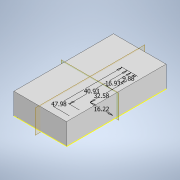
# Autodesk Inventor part: Micro-controller mount
Saved by Autodesk Inventor 2021 (Build 250183000, 183)
## iProperties
Created: 2020-08-19
Part Number: Micro-controller mount
Material: Generic
Document SubType Name: Modeling
Designer: zackh
Density: 1 g/cm^3
Appearance: Default
Author: zackh
Autodesk Inventor part; units mm, degrees
ref_plane "YZ Plane" through (0, 0, 0) normal (1, 0, 0) x (0, 1, 0)
ref_plane "XZ Plane" through (0, 0, 0) normal (0, 1, 0) x (-1, 0, 0)
ref_plane "XY Plane" through (0, 0, 0) normal (0, 0, 1) x (1, 0, 0)
sketch "Sketch1" plane through (0, 0, 0) normal (0, 1, 0) x (-1, 0, 0)
  line L0 (0, 0) -> (37, 0)
  line L1 (37, 0) -> (37, -70)
  line L2 (37, -70) -> (0, -70)
  line L3 (0, -70) -> (0, 0)
  dimension "d0" = 70
  dimension "d1" = 37
  constraints: 8 end point, 2 parallel, 1 horizontal, 1 perpendicular
  measures "d0" distance of L0.end L1.end
  measures "d1" distance of L1.end L2.end
extrude "Extrusion1" add sketch "Sketch1" along normal blind 15
sketch "Sketch2" plane through (0, 0, 0) normal (0, -1, 0) x (1, 0, 0)
  line L0 (-37, 0) -> (0, 0) projected
  line L1 (-18.5, 0) -> (-18.5, -70) construction
  line L2 (0, -70) -> (-37, -70) projected
  line L3 (0, 0) -> (0, -70) projected
  line L4 (0, -35) -> (-37, -35) construction
  line L5 (-37, -70) -> (-37, 0) projected
  line L6 (-2.28, 0) -> (-2.28, -70) construction
  line L7 (-34.72, 0) -> (-34.72, -70) construction
  line L8 (0, -67.58) -> (-35, -67.58) construction
  line L9 (0, -2.42) -> (-35, -2.42) construction
  line L10 (0, -57.7) -> (-35, -57.7) construction
  line L11 (0, -50.65) -> (-35, -50.65) construction
  line L12 (0, -26.65) -> (-35, -26.65) construction
  line L13 (0, -19.6) -> (-35, -19.6) construction
  point P0 (-17.5, -57.7)
  point P1 (-17.5, -50.65)
  point P2 (-17.5, -26.65)
  point P3 (-17.5, -19.6)
  dimension "d4" = 16.22
  dimension "d5" = 32.58
  dimension "d6" = 9.88
  dimension "d7" = 16.93
  dimension "d8" = 40.93
  dimension "d9" = 47.98
  constraints: 20 end point, 8 midpoint, 6 parallel, 4 symmetric about line
  measures "d4" distance between parallel lines of L1 L6
  measures "d5" distance between parallel lines of L4 L8
  measures "d6" distance between parallel lines of L8 L10
  measures "d7" distance between parallel lines of L8 L11
  measures "d8" distance between parallel lines of L8 L12
  measures "d9" distance between parallel lines of L8 L13
hole "Hole1" at (-17.5, 0, -57.7) at (-17.5, 0, -26.65) direction (0, 1, 0) diameter 2.459 depth 10 tip angle 118 thread size "M3x0.5" class "6H" standard "ANSI Metric M Profile"
hole "Hole2" at (-17.5, 0, -50.65) at (-17.5, 0, -19.6) direction (0, 1, 0) diameter 3.4587 depth 10 tip angle 118 thread size "M4x0.5" class "6H" standard "ANSI Metric M Profile"
ref_plane "Work Plane1" through (-18.5, 0, 0) normal (1, 0, 0) x (0, 0, -1)
ref_plane "Work Plane2" through (0, 0, -35) normal (0, 0, -1) x (-1, 0, 0)
body "Solid1"
